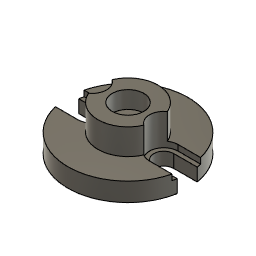
6432106821_SEC_20 (Autodesk Fusion 360 design; units mm, degrees)
Autodesk Fusion 360 part; units mm, degrees
sketch "Sketch1" plane through (0, 0, 0) normal (0, 1, 0) x (1, 0, 0)
  circle A0 centre (0, 0) radius 42
  dimension "d1" = 84
  constraint coincident A0.centre origin
  measures "d1" diameter of A0
extrude "Extrude1" add sketch "Sketch1" along normal blind 13
sketch "Sketch2" plane through (0, 13, 0) normal (0, 1, 0) x (-1, 0, 0)
  circle A0 centre (0, 0) radius 42
sketch "Sketch3" plane through (0, 13, 0) normal (0, 1, 0) x (-1, 0, 0)
  line L0 (0, 0) -> (25, 0) construction
  line L1 (0, 0) -> (-25, 0) construction
  line L2 (-25, 0) -> (-25, 11) construction
  line L3 (-25, 11) -> (-25, -10) construction
  line L4 (-25, -10) -> (-40.3348, -10)
  line L5 (-25, 10) -> (-40.5961, 10)
  arc A0 (-25, -10) -> (-25, 10) centre (-25, 0) ccw
  line L6 (-25, -7) -> (-42.662, -7)
  arc A1 (-25, -7) -> (-25, 7) centre (-25, 0) ccw
  line L7 (-25, 7) -> (-45, 7)
  line L8 (-40.3348, -10) -> (-41.543, -10)
  line L9 (-41.543, -10) -> (-46, -10)
  line L10 (-46, -10) -> (-49, 1)
  line L11 (-49, 1) -> (-46.5662, 10.0079)
  line L12 (-46.5662, 10.0079) -> (-40.5961, 10)
  line L13 (-42.662, -7) -> (-45, 7)
  line L14 (0, -45) -> (0, 45) construction
  arc A2 (25, 10) -> (25, -10) centre (25, 0) ccw
  arc A3 (25, 7) -> (25, -7) centre (25, 0) ccw
  line L15 (25, 7) -> (45, 7)
  line L16 (25, 10) -> (40.5961, 10)
  line L17 (46.5662, 10.0079) -> (40.5961, 10)
  line L18 (49, 1) -> (46.5662, 10.0079)
  line L19 (46, -10) -> (49, 1)
  line L20 (25, -10) -> (40.3348, -10)
  line L21 (41.543, -10) -> (46, -10)
  line L22 (42.662, -7) -> (45, 7)
  line L23 (25, -7) -> (42.662, -7)
  line L24 (40.3348, -10) -> (41.543, -10)
  circle A4 centre (0, 0) radius 21
  circle A5 centre (0, 0) radius 11
  circle A6 centre (0, 0) radius 5
  dimension "d4" = 25
  dimension "d5" = 25
  dimension "d7" = 20
  dimension "d8" = 14
  dimension "d13" = 42
  dimension "d14" = 22
  dimension "d15" = 10
  constraint horizontal L0
  constraint parallel L0 L1
  constraint coincident L1.end L2.start
  constraint perpendicular L1 L2
  constraint perpendicular L1 L3
  constraint coincident L3 L4.start
  constraint tangent L4 A0
  constraint coincident L3 L5.start
  constraint tangent L5 A0
  constraint coincident L3 L6.start
  constraint tangent L6 A1
  constraint coincident L2 A1.end
  constraint tangent A1 L7
  constraint parallel L4 L9
  constraint parallel L3 L14
  constraint symmetric L3.end L14 A2.end
  constraint symmetric L4.end L14 L20.end
  constraint symmetric L5.start L14 A2.start
  constraint symmetric L5.end L14 L16.end
  constraint symmetric A0 L14 A2
  constraint symmetric L6.start L14 A3.end
  constraint symmetric A1.end L14 A3.start
  constraint symmetric A1 L14 A3
  constraint symmetric L7.end L14 L15.end
  constraint symmetric L6.end L14 L22.start
  constraint symmetric L8.end L14 L21.start
  constraint symmetric L9.end L14 L19.start
  constraint symmetric L10.end L14 L18.start
  constraint symmetric L11.end L14 L17.start
  constraint coincident L0.start L1.start
  constraint concentric A5 A6
  measures "d4" distance of L0.start L0.end
  measures "d5" distance of L0.start L1.end
  measures "d7" diameter of A0
  measures "d8" diameter of A1
  measures "d13" diameter of A4
  measures "d14" diameter of A5
  measures "d15" diameter of A6
extrude "Extrude4" cut sketch "Sketch3" against normal blind 4 contours L4 L5 A0 L6 A1 L7 L8 L9 L10 L11 L12 L13 A4 | A0 A1 A4 | A2 A3 L15 L16 L17 L18 L19 L20 L21 L22 L23 L24 A4 | A2 A3 A4
extrude "Extrude5" cut sketch "Sketch3" against normal blind 13 contours A1 A4 | L6 A1 L7 L13 A4 | A3 L15 L22 L23 A4 | A3 A4
extrude "Extrude6" cut sketch "Sketch3" against normal blind 13 contours A6
extrude "Extrude7" add sketch "Sketch3" along normal blind 6 contours A5
extrude "Extrude8" add sketch "Sketch3" along normal blind 18 contours A0 A2 A4
